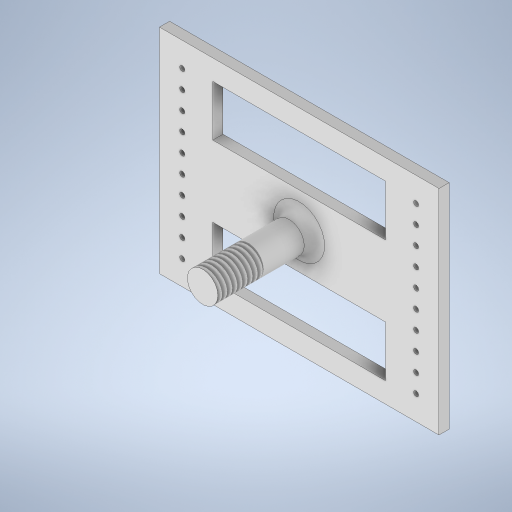
# Autodesk Inventor part: Soporte
Saved by Autodesk Inventor 2023 (Build 270158000, 158)
## iProperties
Created: 2023-08-19
Part Number: Soporte
Material: Generic
Document SubType Name: Modeling
Designer: swimm
Density: 1 g/cm^3
Appearance: Default
Author: swimm
Autodesk Inventor part; units mm, degrees
ref_plane "YZ Plane" through (0, 0, 0) normal (1, 0, 0) x (0, 1, 0)
ref_plane "XZ Plane" through (0, 0, 0) normal (0, 1, 0) x (-1, 0, 0)
ref_plane "XY Plane" through (0, 0, 0) normal (0, 0, 1) x (1, 0, 0)
sketch "Sketch1" plane through (0, 0, 0) normal (0, 0, 1) x (1, 0, 0)
  line L0 (-13.75, -10.5) -> (13.75, -10.5)
  line L1 (13.75, -10.5) -> (13.75, 10.5)
  line L2 (13.75, 10.5) -> (-13.75, 10.5)
  line L3 (-13.75, 10.5) -> (-13.75, -10.5)
  line L4 (-13.75, -10.5) -> (13.75, 10.5) construction
  line L5 (13.75, -10.5) -> (-13.75, 10.5) construction
  line L6 (-8.5, 8.5) -> (8.5, 8.5)
  line L7 (8.5, 8.5) -> (8.5, 3.5)
  line L8 (8.5, 3.5) -> (-8.5, 3.5)
  line L9 (-8.5, 3.5) -> (-8.5, 8.5)
  line L10 (-8.5, 8.5) -> (8.5, 3.5) construction
  line L11 (8.5, 8.5) -> (-8.5, 3.5) construction
  line L12 (-19.25, 0) -> (19.25, 0) construction
  line L13 (-8.5, -8.5) -> (8.5, -8.5)
  line L14 (8.5, -8.5) -> (8.5, -3.5)
  line L15 (8.5, -3.5) -> (-8.5, -3.5)
  line L16 (-8.5, -3.5) -> (-8.5, -8.5)
  line L17 (0, -14.7) -> (0, 14.7) construction
  circle A0 centre (0, 0) radius 1.5
  point P0 (0, 6)
  point P1 (8.5, 6)
  point P2 (11.5, -8.1)
  point P3 (11.5, -6.3)
  point P4 (11.5, -4.5)
  point P5 (11.5, -0.9)
  point P6 (11.5, -2.7)
  point P7 (11.5, 8.1)
  point P8 (11.5, 6.3)
  point P9 (11.5, 4.5)
  point P10 (11.5, 0.9)
  point P11 (11.5, 2.7)
  point P12 (-11.5, -8.1)
  point P13 (-11.5, -6.3)
  point P14 (-11.5, -4.5)
  point P15 (-11.5, -0.9)
  point P16 (-11.5, -2.7)
  point P17 (-11.5, 8.1)
  point P18 (-11.5, 6.3)
  point P19 (-11.5, 4.5)
  point P20 (-11.5, 2.7)
  point P21 (-11.5, 0.9)
  dimension "d0" = 21
  dimension "d1" = 27.5
  dimension "d28" = 17
  dimension "d29" = 5
  dimension "d30" = 2
  dimension "d31" = 1.8
  dimension "d32" = 1.8
  dimension "d33" = 1.8
  dimension "d34" = 1.8
  dimension "d35" = 0.9
  dimension "d36" = 2.25
  dimension "d44" = 3
  constraints: 32 end point, 19 symmetric about line, 5 midpoint, 4 parallel, 4 vertical alignment, 2 horizontal, 2 perpendicular, 1 centre point, 1 coincident, 1 point on line
  measures "d0" distance of L0.end L1.end
  measures "d1" distance of L1.end L2.end
  measures "d28" distance of L6.start L6.end
  measures "d29" distance of L6.end L7.end
  measures "d30" distance between parallel lines of L6 L2
  measures "d31" distance of point (11.5, -6.3) point (11.5, -8.1)
  measures "d32" distance of point (11.5, -6.3) point (11.5, -4.5)
  measures "d33" distance of point (11.5, -4.5) point (11.5, -2.7)
  measures "d34" distance of point (11.5, -2.7) point (11.5, -0.9)
  measures "d35" distance from line of point (11.5, -0.9) L12
  measures "d36" distance from line of L1 point (11.5, -8.1)
  measures "d44" diameter of A0
extrude "Extrusion1" add sketch "Sketch1" against normal blind 1 contours L3 L2 L1 L0 | A0
hole "Hole2" at (11.5, -8.1, 0) at (11.5, -6.3, 0) at (11.5, -4.5, 0) at (11.5, -0.9, 0) at (11.5, -2.7, 0) at (11.5, 8.1, 0) at (11.5, 6.3, 0) at (11.5, 4.5, 0) at (11.5, 2.7, 0) at (11.5, 0.9, 0) at (-11.5, 8.1, 0) at (-11.5, 6.3, 0) at (-11.5, 4.5, 0) at (-11.5, 2.7, 0) at (-11.5, 0.9, 0) at (-11.5, -0.9, 0) at (-11.5, -2.7, 0) at (-11.5, -4.5, 0) at (-11.5, -6.3, 0) at (-11.5, -8.1, 0) direction (0, 0, -1) diameter 0.5 end through all
extrude "Extrusion3" add sketch "Sketch1" along normal blind 9.5 contours A0
thread "Thread3" size "M3x0.5" class "6g" standard "ANSI Metric M Profile" length 4.5
fillet "Fillet3" radius 1 1 edges at (-1.5, 0, 0)
body "Solid1"
